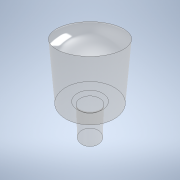
# Autodesk Inventor part: light
Saved by Autodesk Inventor 2020.1 (Build 241239000, 239)
## iProperties
Created: 2019-07-23
Part Number: light
Material: Generic
Document SubType Name: Modeling
Designer: njk024
Density: 1 g/cm^3
Appearance: Default
Author: njk024
Autodesk Inventor part; units mm, degrees
ref_plane "YZ Plane" through (0, 0, 0) normal (1, 0, 0) x (0, 1, 0)
ref_plane "XZ Plane" through (0, 0, 0) normal (0, 1, 0) x (-1, 0, 0)
ref_plane "XY Plane" through (0, 0, 0) normal (0, 0, 1) x (1, 0, 0)
sketch "Sketch1" plane through (0, 0, 0) normal (0, 0, 1) x (1, 0, 0)
  arc A0 (41, -9.8813) -> (0, 0) centre (0, -90) ccw
  line L0 (0, 0) -> (0, -90) construction
  line L1 (0, -90) -> (18.2247, -90) construction
  line L2 (41, -9.8813) -> (41, -90)
  line L3 (41, -90) -> (0, -90)
  line L4 (0, 0) -> (0, -90)
  dimension "d0" = 90
  dimension "d2" = 41
  constraints: 10 end point, 2 perpendicular, 2 point on circle, 1 centre point, 1 collinear, 1 horizontal, 1 point on line, 1 vertical
  measures "d0" distance from line of L1 L0.start
  measures "d2" distance between parallel lines of L2 L0
revolve "Revolution1" add sketch "Sketch1" angle 360 about axis through (0, 0, 0) along (0, -1, 0)
sketch "Sketch2" plane through (0, -90, 0) normal (0, -1, 0) x (1, 0, 0)
  circle A0 centre (0, 0) radius 16.5
  dimension "d4" = 33
  constraints: 1 centre point, 1 coincident
  measures "d4" diameter of A0
extrude "Extrusion1" add sketch "Sketch2" along normal blind 59
fillet "Fillet1" radius 5 1 edges at (-16.5, -90, 0)
body "Solid1"
